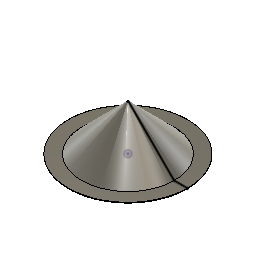
electrode puck v2 assembly v12 (Autodesk Fusion 360 archive; units mm, degrees)
design "electrode v2"
Autodesk Fusion 360 part; units mm, degrees
note: some values were not read from the file. Set by a fixed rule: the direction of a hole.
sketch "Sketch1" plane through (0, 0, 0) normal (0, 0, 1) x (1, 0, 0)
  line L0 (0.0652, 3.4348) -> (3.5, 0)
  line L1 (3.5, 0) -> (4.5, 0)
  line L2 (0.0298, 3.3994) -> (3.4793, -0.05)
  line L3 (3.4793, -0.05) -> (4.5, -0.05)
  line L4 (0.0652, 3.4348) -> (0.0298, 3.3994)
  line L5 (4.5, -0.05) -> (4.5, 0)
  dimension "d1" = 3.5
  dimension "d2" = 1
  dimension "d3" = 45
  dimension "d4" = 0.05
  constraint horizontal L1
  constraint horizontal origin L0.end
  constraint perpendicular L1 L5
  measures "d1" distance of origin L0.end
  measures "d2" distance of L0.end L1.end
  measures "d3" angle of L0 L1
revolve "Revolve1" add sketch "Sketch1" angle 360 about axis through (0, 1.75, 0) along (0, 1, 0)

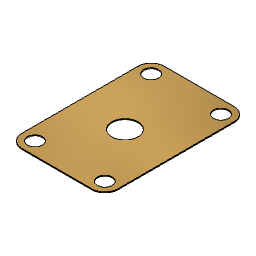
design "front cover"
Autodesk Fusion 360 part; units mm, degrees
sketch "Sketch1" plane through (0, 0, 0) normal (0, 1, 0) x (1, 0, 0)
  line L0 (0, 0) -> (11, 0)
  line L1 (11, 0) -> (11, -16.3)
  line L2 (11, -16.3) -> (0, -16.3)
  line L3 (0, -16.3) -> (0, 0)
  line L4 (1.5, -14.8) -> (1.5, -1.5) construction
  line L5 (1.5, -1.5) -> (9.5, -1.5) construction
  line L6 (9.5, -1.5) -> (9.5, -14.8) construction
  line L7 (9.5, -14.8) -> (1.5, -14.8) construction
  circle A0 centre (5.5, -8.5) radius 1.5
  line L8 (5.5, -14.8) -> (5.5, -8.5) construction
  point P0 (1.5, -1.5)
  point P1 (9.5, -1.5)
  point P2 (9.5, -14.8)
  point P3 (1.5, -14.8)
  dimension "d1" = 16.3
  dimension "d2" = 11
  dimension "d3" = 1.5
  dimension "d4" = 6.3
  dimension "d5" = 3
  constraint horizontal L0
  constraint vertical L1
  constraint horizontal L2
  constraint vertical L3
  constraint coincident L0.start L3.end
  constraint coincident P0 L4.end
  constraint coincident P1 L5.end
  constraint coincident P2 L6.end
  constraint coincident P3 L4.start
  constraint midpoint L7 L8.start
  constraint coincident A0.centre L8.end
  constraint vertical L8
  measures "d1" distance of L0.start L2.end
  measures "d2" distance of L0.start L0.end
  measures "d4" distance of L7 A0.centre
  measures "d5" diameter of A0
extrude "Extrude1" add sketch "Sketch1" along normal blind 0.1
hole "Hole1" at (1.5, 0, 14.8) at (1.5, 0, 1.5) at (9.5, 0, 1.5) at (9.5, 0, 14.8) direction (0, 1, 0) diameter 1.7 depth 12 tip angle 118
fillet "Fillet1" radius 1.5 4 edges at (11, 0.05, 16.3) (0, 0.05, 16.3) (0, 0.05, 0) (11, 0.05, 0)
equation "d1 = 11.3 mm + 5 mm"
equation "d2 = 8 mm + 3 mm"

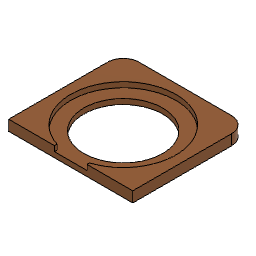
design "electrode puck v2 insulation"
Autodesk Fusion 360 part; units mm, degrees
sketch "Sketch1" plane through (0, 0, 0) normal (0, 1, 0) x (1, 0, 0)
  line L0 (0, 0) -> (12, 0)
  line L1 (12, 0) -> (12, -11)
  line L2 (12, -11) -> (0, -11)
  line L3 (0, -11) -> (0, 0)
  circle A0 centre (6, -6) radius 3.75
  line L4 (6, -11) -> (6, -6) construction
  line L5 (1, -11) -> (1, -1)
  line L6 (1, -1) -> (11, -1)
  line L7 (11, -1) -> (11, -11)
  circle A1 centre (6, -6) radius 5
  line L8 (4.45, -10.7537) -> (4.45, -11)
  line L9 (7.55, -10.7537) -> (7.55, -11)
  arc A2 (3.299, -11) -> (0.701, -11) centre (2, -11.75) ccw
  dimension "d1" = 12
  dimension "d2" = 11
  dimension "d3" = 5
  dimension "d4" = 7.5
  dimension "d5" = 1
  dimension "d11" = 10
  dimension "d12" = 3.1
  dimension "d14" = 1.5
  dimension "d15" = 4
  dimension "d16" = 0.75
  constraint horizontal L0
  constraint vertical L1
  constraint horizontal L2
  constraint vertical L3
  constraint coincident L0.start L3.end
  constraint midpoint L2 L4.start
  constraint coincident A0.centre L4.end
  constraint perpendicular L2 L4
  constraint concentric A0 A1
  constraint coincident A1 L8.start
  constraint coincident L2 L8.end
  constraint perpendicular L2 L8
  constraint coincident A1 L9.start
  constraint coincident L2 L9.end
  constraint perpendicular L2 L9
  constraint symmetric L4 L8 L9
  constraint coincident L2 A2.start
  constraint coincident L2 A2.end
  measures "d1" distance of L1.end L2.end
  measures "d2" distance of L0.end L1.end
  measures "d3" distance of L2 A0.centre
  measures "d4" diameter of A0
  measures "d11" diameter of A1
  measures "d12" distance of L8 L9
  measures "d14" radius of A2
  measures "d15" distance of L4 A2.centre
  measures "d16" distance of L2 A2.centre
extrude "Extrude1" add sketch "Sketch1" along normal blind 1 contours L0 L1 L2 L3 L5 L6 L7 A2 | L2 L5 A2 | L2 L7 A1 L9 | L2 L5 A2 | L2 L5 A1 L8 A2 | L6 L7 A1 | L5 L6 A1
extrude "Extrude2" add sketch "Sketch1" along normal blind 0.5 contours L2 L7 A1 L9 | L2 L5 A2 | L2 L5 A1 L8 A2 | L2 A1 L9 | L6 L7 A1 | A1 | L5 L6 A1 | L2 A1 L8 picked at (2.4911, -10.9389)
fillet "Fillet1" radius 1.5 2 edges at (12, 0.5, 0) (0, 0.5, 0)
move_face "OffsetFaces1" offset -0.1 3 faces at (12, 0.3333, 4.6667) (4.5, 0.3333, 0) (0, 0.3333, 7.8333)

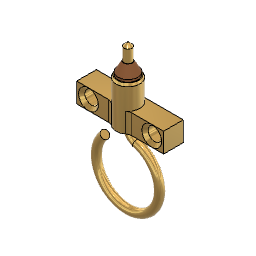
design "electrode puck v2 connector"
Autodesk Fusion 360 part; units mm, degrees
sketch "Sketch1" plane through (0, 0, 0) normal (0, 1, 0) x (1, 0, 0)
  circle A0 centre (0, 0) radius 0.5
  circle A1 centre (0, 0) radius 1.25
  circle A2 centre (0, 0) radius 1.5
  line L0 (-5.5, 1.5) -> (5.5, 1.5)
  line L1 (5.5, 1.5) -> (5.5, -1)
  line L2 (5.5, -1) -> (1.118, -1)
  line L3 (-1.118, -1) -> (-5.5, -1)
  line L4 (-5.5, -1) -> (-5.5, 1.5)
  line L5 (0, -20) -> (0, -2.5) construction
  dimension "d1" = 1
  dimension "d2" = 2.5
  dimension "d3" = 3
  dimension "d4" = 2.5
  dimension "d17" = 11
  constraint coincident A0.centre A1.centre
  constraint horizontal L0
  constraint perpendicular L0 L1
  constraint perpendicular L1 L2
  constraint perpendicular L0 L4
  constraint perpendicular L3 L4
  constraint tangent A2 L0
  constraint collinear L2 L3
  constraint coincident A2 L2.end
  constraint coincident A2 L3.start
  measures "d1" diameter of A0
  measures "d2" diameter of A1
  measures "d3" diameter of A2
  measures "d4" distance of L0.end L1.end
  measures "d17" distance of L1 L4
extrude "Extrude1" add sketch "Sketch1" along normal blind 2.5 contours A2 | A2 L0 L3 L4 | A2 L0 L1 L2 makes body 1
extrude "Extrude2" add sketch "Sketch1" along normal blind 5.5 contours A2 bodies 1
fillet "Fillet1" radius 1 2 edges at (1.118, 1.25, 1) (-1.118, 1.25, 1) on bodies 1
extrude "Extrude3" add sketch "Sketch1" along normal blind 7 separate body contours A1 makes body 2
extrude "Extrude4" add sketch "Sketch1" along normal blind 9 separate body contours A0 makes body 3
chamfer "Chamfer1" distance 0.4 angle 45 1 edges at (-0.4662, 9, 0.1808) on bodies 3
sketch "Sketch2" plane through (0, 0, 0) normal (0, 0, 1) x (1, 0, 0)
  arc A0 (0, 0) -> (1.0909, -1.4431) centre (1.5, 0) ccw
  arc A1 (-2.927, -2.5652) -> (1.0909, -1.4431) centre (0, -5.2915) ccw
  dimension "d19" = 1.5
  dimension "d20" = 4
  constraint tangent A0 A1
  constraint coincident A0.start origin
  constraint horizontal A0.centre A0.start
  constraint vertical A1.centre A0.start
  measures "d19" radius of A0
  measures "d20" radius of A1
sweep "Sweep1" add profiles "Sketch1" path "Sketch2" along A0 A1 section 1 contours A0 bodies 3
sketch "Sketch3" plane through (0, 0, 1) normal (0, 0, 1) x (-1, 0, 0)
  line L0 (-5.5, 0) -> (5.5, 0)
  line L1 (0, 1.75) -> (0, 22.5) construction
  line L2 (-5.5, -1.25) -> (5.5, -1.25) construction
  line L3 (-1.5, -2.5) -> (-1.5, 0)
  line L4 (-1.5, 0) -> (-5.5, 0)
  line L5 (-5.5, 0) -> (-5.5, -2.5)
  line L6 (-5.5, -2.5) -> (-1.5, -2.5)
  point P0 (-4, -1.25)
  point P1 (4, -1.25)
  dimension "d27" = 8
  constraint symmetric P0 P1 L1
  constraint coincident P0 L2
  constraint midpoint L2.start L5
  constraint horizontal L2
  measures "d27" distance of P0 P1
hole "Hole1" at (4, 1.25, 1) at (-4, 1.25, 1) direction (0, 0, -1) diameter 1.7 depth 6 tip angle 118 countersink diameter 2.5 countersink angle 90 bodies 1
chamfer "Chamfer2" distance 0.7 angle 60 1 edges at (-1.1654, 7, 0.452) measured on face at (0.9935, 7, 0.0869) on bodies 2
chamfer "Chamfer3" distance 0.15 angle 65 1 edges at (-1.3985, 5.5, 0.5424) measured on face at (-1.3264, 5.5, 0.4871) on bodies 1
copy_body "Body->Comp1" bodies 1 removing the originals makes body 4 in component "main gnd"
copy_body "Body->Comp2" bodies 2 removing the originals makes body 5 in component "dielectric"
copy_body "Body->Comp3" bodies 3 removing the originals makes body 6 in component "conductor"
component "main gnd" placed x (1, 0, 0) y (0, 1, 0) z (0, 0, 1) at (0, 0, 0)
component "dielectric" placed x (1, 0, 0) y (0, 1, 0) z (0, 0, 1) at (0, 0, 0)
component "conductor" placed x (1, 0, 0) y (0, 1, 0) z (0, 0, 1) at (0, 0, 0)
named bodies: "main gnd", "dielectric", "conductor"
